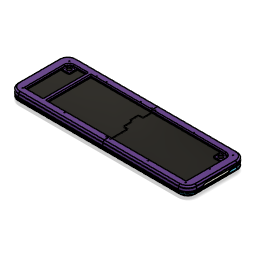
Future Keyboard 2 (Autodesk Fusion 360 design; units mm, degrees)
Autodesk Fusion 360 part; units mm, degrees
note: some values were not read from the file. Chosen so that the rebuilt part matches the saved one: which bodies a step acts on; which face or edge a step refers to; where a step ends. Set by a fixed rule: which sketch regions a step uses.
(part 1 of 2)
sketch "Sketch1" plane through (0, 0, 0) normal (0, 1, 0) x (1, 0, 0)
  arc A0 (365.425, 0) -> (368.425, 3) centre (365.425, 3) ccw
  arc A1 (179.45, 67.614) -> (181.45, 65.614) centre (181.45, 67.614) ccw
  arc A2 (184.212, 48.554) -> (186.212, 46.554) centre (186.212, 48.554) ccw
  circle A3 centre (160.955, 107.775) radius 1.1
  circle A4 centre (363.725, 3.65) radius 1.1
  line L0 (365.425, 111.675) -> (3, 111.675)
  arc A5 (3, 111.675) -> (0, 108.675) centre (3, 108.675) ccw
  circle A6 centre (97.24, 4) radius 1.1
  circle A7 centre (364.375, 55.975) radius 1.1
  line L1 (3, 0) -> (365.425, 0)
  line L2 (368.425, 3) -> (368.425, 108.675)
  circle A8 centre (197.837, 4) radius 1.1
  line L3 (184.212, 63.614) -> (184.212, 48.554)
  line L4 (186.212, 46.554) -> (191.737, 46.554)
  circle A9 centre (184.98, 107.775) radius 1.1
  line L5 (181.45, 65.614) -> (182.212, 65.614)
  circle A10 centre (63.622, 107.775) radius 1.1
  arc A11 (0, 3) -> (3, 0) centre (3, 3) ccw
  arc A12 (181.45, 84.67) -> (179.45, 82.67) centre (181.45, 82.67) ccw
  line L6 (0, 108.675) -> (0, 3)
  circle A13 centre (85.74, 107.775) radius 1.1
  line L7 (186.975, 84.67) -> (181.45, 84.67)
  circle A14 centre (280.925, 4.15) radius 1.1
  arc A15 (184.212, 63.614) -> (182.212, 65.614) centre (182.212, 63.614) ccw
  line L8 (179.45, 82.67) -> (179.45, 67.614)
  arc A16 (193.737, 44.554) -> (191.737, 46.554) centre (191.737, 44.554) ccw
  circle A17 centre (193.075, 107.675) radius 1.1
  circle A18 centre (278.425, 107.625) radius 1.1
  circle A19 centre (4.7, 4.7) radius 1.1
  circle A20 centre (363.825, 107.715) radius 1.1
  arc A21 (368.425, 108.675) -> (365.425, 111.675) centre (365.425, 108.675) ccw
  arc A22 (186.975, 84.67) -> (188.975, 86.67) centre (186.975, 86.67) ccw
  circle A23 centre (4.7, 106.975) radius 1.1
  line L9 (188.975, 111.675) -> (188.975, 86.67)
  line L10 (193.737, 44.554) -> (193.737, 0)
  circle A24 centre (189.74, 4) radius 1.1
  point P0 (368.425, 111.675)
  point P1 (0, 111.675)
  point P2 (184.212, 46.554)
  point P3 (188.975, 84.67)
  point P4 (179.45, 83.9809)
  point P5 (179.45, 65.614)
  point P6 (184.212, 58.87)
  dimension "d1" = 368.425
  dimension "d2" = 111.675
  dimension "d3" = 3
  dimension "d43" = 188.975
  dimension "d45" = 179.45
  dimension "d46" = 184.212
  dimension "d47" = 193.737
  dimension "d48" = 27.005
  dimension "d51" = 2
  dimension "d52" = 19.06
  dimension "d53" = 19.056
  dimension "d227" = 4.7
  dimension "d228" = 4.7
  dimension "d229" = 2.2
  dimension "d230" = 4.7
  dimension "d231" = 3.9
  dimension "d232" = 4
  dimension "d233" = 58.922
  dimension "d234" = 22.118
  dimension "d235" = 75.215
  dimension "d236" = 24.025
  dimension "d237" = 92.54
  dimension "d238" = 92.5
  dimension "d239" = 4
  dimension "d240" = 4.1
  dimension "d242" = 89.45
  dimension "d243" = 3.96
  dimension "d244" = 4.6
  dimension "d245" = 4.05
  dimension "d246" = 55.7
  dimension "d247" = 4.7
  dimension "d248" = 3.65
  dimension "d249" = 87.5
  dimension "d250" = 4.15
  dimension "d251" = 4
  dimension "d252" = 4.1
  dimension "d253" = 4.05
  constraint horizontal L1
  constraint vertical L2
  constraint horizontal L0
  constraint vertical L6
  constraint coincident P1 L0
  constraint coincident P1 L6
  constraint tangent L0 A5
  constraint tangent A5 L6
  constraint coincident origin L1
  constraint coincident origin L6
  constraint tangent L1 A11
  constraint tangent A11 L6
  constraint equal A5 A11
  constraint tangent A0 L1
  constraint tangent A0 L2
  constraint equal A0 A5
  constraint coincident P0 L2
  constraint coincident P0 L0
  constraint tangent L2 A21
  constraint tangent L0 A21
  constraint equal A5 A21
  constraint vertical L9
  constraint coincident L9.start L0
  constraint vertical L8
  constraint vertical L3
  constraint coincident L10.end L1
  constraint perpendicular L1 L10
  constraint perpendicular L7 L9
  constraint perpendicular L5 L8
  constraint perpendicular L4 L10
  constraint coincident P4 L8
  constraint tangent A12 L8
  constraint tangent A12 L7
  constraint coincident P3 L9
  constraint coincident P3 L7
  constraint tangent A22 L9
  constraint tangent L7 A22
  constraint equal A12 A22
  constraint coincident P5 L8
  constraint coincident P5 L5
  constraint tangent A1 L8
  constraint tangent A1 L5
  constraint equal A1 A12
  constraint coincident P6 L3
  constraint tangent L3 A15
  constraint tangent L5 A15
  constraint equal A12 A15
  constraint tangent L4 A16
  constraint tangent A16 L10
  constraint equal A12 A16
  constraint coincident P2 L4
  constraint coincident P2 L3
  constraint tangent A2 L4
  constraint tangent A2 L3
  constraint equal A2 A12
  constraint horizontal A13.centre A3.centre
  constraint horizontal A3.centre A9.centre
  constraint horizontal A6.centre A24.centre
  constraint horizontal A13.centre A10.centre
  constraint equal A10 A23
  constraint equal A10 A13
  constraint equal A3 A13
  constraint equal A3 A9
  constraint equal A9 A24
  constraint equal A6 A24
  constraint equal A6 A19
  constraint vertical A23.centre A19.centre
  constraint equal A17 A18
  constraint equal A18 A20
  constraint equal A7 A20
  constraint equal A4 A7
  constraint equal A4 A14
  constraint equal A8 A14
  constraint equal A3 A17
  constraint coincident L1.start L6
  measures "d1" distance of P0 P1
  measures "d2" distance of origin P1
  measures "d3" radius of A5
  measures "d43" distance of L6 L9
  measures "d45" distance of L6 L8
  measures "d46" distance of L3 L6
  measures "d47" distance of L6 L10
  measures "d48" distance of L9.start P3
  measures "d51" radius of A12
  measures "d52" distance of L4 L5
  measures "d53" distance of L5 L7
  measures "d227" distance of A23.centre L6
  measures "d228" distance of A23.centre L0
  measures "d229" diameter of A23
  measures "d230" distance of A19.centre L1
  measures "d231" distance of A10.centre L0
  measures "d232" distance of A6.centre L1
  measures "d233" horizontal distance of A23.centre A10.centre
  measures "d234" distance of A13.centre A10.centre
  measures "d235" distance of A13.centre A3.centre
  measures "d236" distance of A3.centre A9.centre
  measures "d237" horizontal distance of A19.centre A6.centre
  measures "d238" distance of A6.centre A24.centre
  measures "d239" distance of A17.centre L0
  measures "d240" distance of A17.centre L9
  measures "d242" distance of A18.centre L9
  measures "d243" distance of A20.centre L0
  measures "d244" distance of A20.centre L2
  measures "d245" distance of A7.centre L2
  measures "d246" distance of A7.centre L0
  measures "d247" distance of A4.centre L2
  measures "d248" distance of A4.centre L1
  measures "d249" distance of A14.centre L2
  measures "d250" distance of A14.centre L1
  measures "d251" distance of A8.centre L1
  measures "d252" distance of A8.centre L10
  measures "d253" distance of A18.centre L0
sketch "Sketch2" plane through (0, 0, 0) normal (0, 1, 0) x (1, 0, 0)
  line L0 (360, -8.3249) -> (8.425, -8.3249)
  line L1 (-11.575, 11.6751) -> (-11.575, 99.9999)
  line L2 (8.425, 119.9999) -> (360, 119.9999)
  line L3 (380, 99.9999) -> (380, 11.6751)
  arc A0 (8.425, 119.9999) -> (-11.575, 99.9999) centre (8.425, 99.9999) ccw
  arc A1 (-11.575, 11.6751) -> (8.425, -8.3249) centre (8.425, 11.6751) ccw
  arc A2 (360, -8.3249) -> (380, 11.6751) centre (360, 11.6751) ccw
  arc A3 (380, 99.9999) -> (360, 119.9999) centre (360, 99.9999) ccw
  line L4 (365.425, 111.675) -> (3, 111.675) construction
  line L5 (0, 108.675) -> (0, 3) construction
  line L6 (3, 0) -> (365.425, 0) construction
  line L7 (368.425, 3) -> (368.425, 108.675) construction
  line L8 (0, 55.8375) -> (368.425, 55.8375) construction
  line L9 (184.2125, 0) -> (184.2125, 111.675) construction
  line L10 (8.425, 11.6751) -> (360, 99.9999) construction
  line L11 (8.425, 99.9999) -> (360, 11.6751) construction
  point P0 (3, 3)
  point P1 (3, 108.675)
  point P2 (365.425, 108.675)
  point P3 (365.425, 3)
  point P4 (184.2125, 55.8375)
  dimension "d42" = 20
  constraint horizontal L0
  constraint perpendicular L0 L1
  constraint parallel L0 L2
  constraint parallel L1 L3
  constraint tangent L1 A0
  constraint tangent L2 A0
  constraint tangent L0 A1
  constraint tangent L1 A1
  constraint equal A0 A1
  constraint tangent L0 A2
  constraint tangent L3 A2
  constraint equal A0 A2
  constraint tangent L3 A3
  constraint tangent L2 A3
  constraint equal A0 A3
  constraint midpoint L5 L8.start
  constraint midpoint L7 L8.end
  constraint midpoint L6 L9.start
  constraint midpoint L4 L9.end
  constraint coincident A1.centre L10.start
  constraint coincident A3.centre L10.end
  constraint coincident A0.centre L11.start
  constraint coincident A2.centre L11.end
  constraint midpoint L11 P4
  constraint coincident L9 P4
  constraint coincident L8 P4
  measures "d42" radius of A0
extrude "Extrude3" add sketch "Sketch2" along normal blind 6.6 and the other way blind 20 makes body 1
ref_plane "WorkPlane7" through (184.2125, -20, -55.8375) normal (0, -1, 0) x (-1, 0, 0)
sketch "Sketch3" plane through (-11.575, 0, 0) normal (-1, 0, 0) x (0, 0, 1)
  line L0 (-11.6751, -20) -> (-11.6751, 6.6) construction
  line L1 (-11.6751, 6.6) -> (-99.9999, 6.6) construction
  line L2 (-99.9999, 6.6) -> (-99.9999, -20) construction
  line L3 (-99.9999, -20) -> (-11.6751, -20) construction
  line L4 (-99.9999, -20) -> (-99.9999, 6.6) construction
  line L5 (-99.9999, 6.6) -> (-119.9999, 6.6) construction
  line L6 (-119.9999, 6.6) -> (-119.9999, -20) construction
  line L7 (-119.9999, -20) -> (-99.9999, -20) construction
  line L8 (8.3249, -20) -> (8.3249, 6.6) construction
  line L9 (8.3249, 6.6) -> (-11.6751, 6.6) construction
  line L10 (-11.6751, 6.6) -> (-11.6751, -20) construction
  line L11 (-11.6751, -20) -> (8.3249, -20) construction
  line L12 (8.3249, -20) -> (-119.9999, -20)
  line L13 (-119.9999, -20) -> (8.3249, -13.2748)
  line L14 (8.3249, -13.2748) -> (8.3249, -20)
  dimension "d55" = 3
  constraint coincident L8.start L11.end
  constraint coincident L6.end L7.start
  constraint coincident L8 L13.end
  measures "d55" angle of L12 L13
extrude "Extrude4" cut sketch "Sketch3" against normal through all bodies 1
ref_plane "WorkPlane3" through (184.2125, -13.2748, 8.3249) normal (0, -1, 0) x (1, 0, 0)
ref_plane "WorkPlane4" through (184.2125, -10.2748, 8.3249) normal (0, -1, 0) x (1, 0, 0)
sketch "Sketch4" plane through (184.2125, -10.2748, -55.8375) normal (0, -1, 0) x (1, 0, 0)
  arc A0 (-195.7875, -44.1624) -> (-175.7875, -64.1624) centre (-175.7875, -44.1624) ccw
  line L0 (-175.7875, -64.1624) -> (175.7875, -64.1624)
  arc A1 (175.7875, -64.1624) -> (195.7875, -44.1624) centre (175.7875, -44.1624) ccw
  line L1 (195.7875, -44.1624) -> (195.7875, 44.1624)
  arc A2 (195.7875, 44.1624) -> (175.7875, 64.1624) centre (175.7875, 44.1624) ccw
  line L2 (175.7875, 64.1624) -> (-175.7875, 64.1624)
  arc A3 (-175.7875, 64.1624) -> (-195.7875, 44.1624) centre (-175.7875, 44.1624) ccw
  line L3 (-195.7875, 44.1624) -> (-195.7875, -44.1624)
ref_plane "WorkPlane2" through (184.2125, -6.7, -55.8375) normal (1, 0, 0) x (0, 0, -1)
sketch "Sketch5" plane through (184.2125, -13.9511, -55.8375) normal (1, 0, 0) x (0, 0, -1)
  line L0 (-64.1624, 0.6763) -> (64.1624, -6.0489) construction
  line L1 (64.1624, -6.0489) -> (64.1624, 20.5511) construction
  line L2 (64.1624, 20.5511) -> (-64.1624, 20.5511) construction
  line L3 (-64.1624, 20.5511) -> (-64.1624, 0.6763) construction
  line L4 (64.1624, 3.6763) -> (54.9215, -5.5646)
  line L5 (54.9215, -5.5646) -> (54.1703, -19.8984)
  line L6 (54.1703, -19.8984) -> (81.2796, -21.3191)
  line L7 (81.2796, -21.3191) -> (82.539, 2.7132)
  line L8 (82.539, 2.7132) -> (64.1624, 3.6763)
  point P0 (64.1624, 3.6763)
  dimension "d72" = 45
  constraint coincident P0 L4.start
  constraint coincident L0 L4.end
  constraint perpendicular L0 L5
  constraint perpendicular L5 L6
  constraint perpendicular L6 L7
  constraint perpendicular L5 L8
  measures "d72" angle of L1 L4
sweep "Sweep1" cut profiles "Sketch5" path "Sketch4" along L0 A1 L1 A2 L2 A3 L3 A0 section 1 bodies 1
chamfer "Chamfer1" distance 3 angle 45 8 edges at (-5.7171, 6.6, 2.4671) (184.2125, 6.6, 8.3249) (374.1421, 6.6, 2.4671) (380, 6.6, -55.8375) (374.1421, 6.6, -114.1421) (184.2125, 6.6, -119.9999) (-5.7171, 6.6, -114.1421) (-11.575, 6.6, -55.8375) on bodies 1
ref_plane "WorkPlane5" through (184.2125, 3.6, -55.8375) normal (0, 1, 0) x (1, 0, 0)
ref_plane "WorkPlane6" through (184.2125, -3.3374, -55.8375) normal (0, 1, 0) x (1, 0, 0)
sketch "Sketch6" plane through (0, 0, 0) normal (0, 1, 0) x (1, 0, 0)
  line L0 (8, 85.1196) -> (26.3429, 85.1196)
  line L1 (17.525, 103.4625) -> (46.1, 103.4625)
  line L2 (8, 93.9375) -> (8, 103.4625) construction
  circle A0 centre (17.525, 93.9375) radius 4.5
  line L3 (27.05, 84.4125) -> (27.05, 103.4625) construction
  line L4 (46.1, 8.2125) -> (8, 8.2125)
  line L5 (27.05, 84.4125) -> (8, 103.4625) construction
  arc A1 (17.525, 103.4625) -> (8, 93.9375) centre (17.525, 93.9375) ccw
  line L6 (8, 103.4625) -> (17.525, 103.4625) construction
  line L7 (8, 84.4125) -> (27.05, 103.4625) construction
  line L8 (360.425, 8.2125) -> (55.625, 8.2125)
  line L9 (55.625, 103.4625) -> (350.9, 103.4625)
  arc A2 (360.425, 93.9375) -> (350.9, 103.4625) centre (350.9, 93.9375) ccw
  circle A3 centre (350.9, 93.9375) radius 4.5
  line L10 (341.375, 103.4625) -> (341.375, 84.4125) construction
  line L11 (350.9, 103.4625) -> (360.425, 103.4625) construction
  line L12 (360.425, 103.4625) -> (360.425, 93.9375) construction
  line L13 (342.0821, 103.4625) -> (342.0821, 85.1196)
  circle A4 centre (350.9, 93.9375) radius 7.5 construction
  line L14 (341.375, 103.4625) -> (360.425, 84.4125) construction
  line L15 (342.0821, 85.1196) -> (360.425, 85.1196)
  line L16 (341.375, 84.4125) -> (360.425, 103.4625) construction
  line L17 (360.425, 93.9375) -> (360.425, 8.2125)
  line L18 (341.375, 84.4125) -> (360.425, 84.4125) construction
  line L19 (55.625, 8.2125) -> (55.625, 103.4625)
  line L20 (8, 84.4125) -> (27.05, 84.4125) construction
  line L21 (46.1, 103.4625) -> (46.1, 8.2125)
  line L22 (8, 8.2125) -> (8, 93.9375)
  line L23 (26.3429, 85.1196) -> (26.3429, 103.4625)
  line L24 (365.425, 111.675) -> (3, 111.675)
  line L25 (0, 108.675) -> (0, 3)
  line L26 (3, 0) -> (365.425, 0)
  line L27 (368.425, 3) -> (368.425, 108.675)
  line L28 (360.425, 51.075) -> (368.425, 51.075) construction
  line L29 (0, 55.8375) -> (8, 55.8375) construction
  line L30 (184.2125, 0) -> (184.2125, 8.2125) construction
  line L31 (184.2125, 111.675) -> (184.2125, 103.4625) construction
  line L32 (24.525, 100.9375) -> (10.525, 100.9375)
  line L33 (10.525, 100.9375) -> (10.525, 86.9375)
  line L34 (10.525, 86.9375) -> (24.525, 86.9375)
  line L35 (24.525, 86.9375) -> (24.525, 100.9375)
  line L36 (24.525, 100.9375) -> (10.525, 86.9375) construction
  line L37 (10.525, 100.9375) -> (24.525, 86.9375) construction
  line L38 (357.9, 100.9375) -> (343.9, 100.9375)
  line L39 (343.9, 100.9375) -> (343.9, 86.9375)
  line L40 (343.9, 86.9375) -> (357.9, 86.9375)
  line L41 (357.9, 86.9375) -> (357.9, 100.9375)
  line L42 (357.9, 100.9375) -> (343.9, 86.9375) construction
  line L43 (343.9, 100.9375) -> (357.9, 86.9375) construction
  point P0 (191.1727, 8.2125)
  point P1 (8, 59.175)
  point P2 (360.425, 54.8137)
  point P3 (17.525, 93.9375)
  point P4 (350.9, 93.9375)
  dimension "d185" = -1
  dimension "d186" = -1
  dimension "d7" = 304.8
  dimension "d8" = 95.25
  dimension "d9" = 38.1
  dimension "d10" = 9.525
  dimension "d176" = 19.05
  dimension "d177" = 15
  dimension "d180" = 19.05
  dimension "d181" = 9
  dimension "d182" = 9
  dimension "d87" = 1
  dimension "d198" = 14
  dimension "d199" = 14
  constraint coincident P0 L8
  constraint equal L19 L21
  constraint collinear L1 L9
  constraint coincident P1 L22
  constraint coincident L10.start L9
  constraint perpendicular L9 L10
  constraint coincident L14.end L17
  constraint perpendicular L17 L18
  constraint equal L10 L18
  constraint midpoint P4 L16
  constraint concentric A2 A4
  constraint tangent L9 A2
  constraint coincident P2 L17
  constraint tangent L1 A1
  constraint tangent A1 L22
  constraint equal A1 A2
  constraint coincident L7.start L22
  constraint perpendicular L20 L22
  constraint coincident L3.end L1
  constraint perpendicular L1 L3
  constraint equal L3 L20
  constraint concentric A3 A4
  constraint concentric A0 A1
  constraint parallel L0 L20
  constraint parallel L3 L23
  constraint parallel L10 L13
  constraint parallel L15 L18
  constraint midpoint L17 L28.start
  constraint coincident L27 L28.end
  constraint perpendicular L27 L28
  constraint midpoint L25 L29.start
  constraint coincident L22 L29.end
  constraint perpendicular L22 L29
  constraint perpendicular L8 L17
  constraint perpendicular L8 L19
  constraint perpendicular L9 L19
  constraint perpendicular L4 L21
  constraint perpendicular L4 L22
  constraint coincident L23.end L1
  constraint coincident L0.start L22
  constraint coincident L0.end L5
  constraint perpendicular L2 L6
  constraint perpendicular L3 L6
  constraint midpoint L26 L30.start
  constraint coincident L8 L30.end
  constraint perpendicular L8 L30
  constraint midpoint L24 L31.start
  constraint coincident L9 L31.end
  constraint perpendicular L9 L31
  constraint equal L30 L31
  constraint parallel L9 L24
  constraint coincident L13.end L16
  constraint coincident L13.start L9
  constraint coincident L15.end L17
  constraint tangent A2 L17
  constraint equal L28 L29
  constraint perpendicular L11 L12
  constraint equal L0 L15
  constraint horizontal L32
  constraint perpendicular L32 L33
  constraint parallel L32 L34
  constraint parallel L33 L35
  constraint coincident L7 L32.start
  constraint coincident L36 P3
  constraint coincident L37 P3
  constraint coincident P3 A0.centre
  constraint horizontal L38
  constraint perpendicular L38 L39
  constraint parallel L38 L40
  constraint parallel L39 L41
  constraint coincident L16 L38.start
  constraint coincident L42 P4
  constraint coincident L43 P4
  constraint coincident P4 A2.centre
  measures "d7" distance of L9.start L11.end
  measures "d8" distance of L9.start L8.end
  measures "d9" distance of L2.end L1.end
  measures "d10" distance of L19 L21
  measures "d176" distance of L10.start L10.end
  measures "d177" diameter of A4
  measures "d180" distance of L3.start L3.end
  measures "d181" diameter of A3
  measures "d182" diameter of A0
  measures "d87" distance of L0.end L3.start
  measures "d198" distance of L32.start L32.end
  measures "d199" distance of L38.start L38.end
extrude "Extrude5" cut sketch "Sketch6" along normal through all contours L0 L1 L4 L21 L22 L23 | L8 L9 L13 L15 L17 L19 bodies 1
extrude "Extrude6" cut sketch "Sketch1" along normal blind 1.6 contours A0 A1 A2 L0 L1 L2 L3 L4 L5 A12 L7 A15 L8 A16 A21 A22 L9 L10 | A1 A2 L0 A5 L1 L3 L4 L5 A11 A12 L6 L7 A15 L8 A16 A22 L9 L10 | A3 | A4 | A6 | A7 | A8 | A9 | A10 | A13 | A14 | A17 | A18 | A19 | A20 | A23 | A24 bodies 1
extrude "Extrude10" add sketch "Sketch1" along normal blind 1.6 separate body makes body 2
extrude "Extrude8" cut sketch "Sketch6" along normal through all contours A0 | A3 bodies 1
extrude "Extrude9" cut sketch "Sketch6" against normal blind 3 from surface at 6.6 contours L0 L1 A1 L22 L23 L32 L33 L34 L35 | A1 L32 L33 L34 L35 | L9 A2 L13 L15 L17 L38 L39 L40 L41 | A2 L38 L39 L40 L41 bodies 1
extrude "Extrude23" cut sketch "Sketch6" along normal blind 1 from surface at 1.6 contours A1 L32 L33 | A1 L32 L33 L34 L35 | A2 L38 L39 L40 L41 | A2 L38 L41 bodies 1
chamfer "Chamfer2" distance 2 angle 45 2 edges at (342.0821, 2.6, -85.1196) (26.3429, 2.6, -85.1196) on bodies 1
chamfer "Chamfer3" distance 2 angle 45 10 edges at (31.8125, 6.6, -103.4625) (8, 6.6, -51.075) (10.7898, 6.6, -100.6727) (46.1, 6.6, -55.8375) (27.05, 6.6, -8.2125) (55.625, 6.6, -55.8375) (203.2625, 6.6, -103.4625) (357.6352, 6.6, -100.6727) (360.425, 6.6, -51.075) (208.025, 6.6, -8.2125) on bodies 1
split "Split1" by plane through (0, 0, 0) normal (0, 1, 0) bodies 1 makes body 3 at (372.1417, 6.6, -68.5375)
shell "Shell1" thickness 5 removed faces 2 at (244.6167, 0, -37.225) at (372.2833, 0, -70.5583) on bodies 1
sketch "Sketch7" plane through (184.2125, -9.2, -55.8375) normal (1, 0, 0) x (0, 0, -1)
  line L0 (159.4764, 5.8626) -> (-230.5357, 5.8626) construction
  line L1 (-60.9965, -4.2407) -> (54.9215, -10.3157) construction
  line L2 (54.9215, -10.3157) -> (64.1624, -1.0748) construction
  line L3 (64.1624, -1.0748) -> (64.1624, 9.2) construction
  line L4 (64.1624, 9.2) -> (59.1624, 9.2) construction
  line L5 (59.1624, 9.2) -> (59.1624, 0.9963) construction
  line L6 (59.1624, 0.9963) -> (52.9601, -5.206) construction
  line L7 (52.9601, -5.206) -> (-58.8181, 0.652) construction
  line L8 (-58.8181, 0.652) -> (-59.1624, 0.9963) construction
  line L9 (-59.1624, 0.9963) -> (-59.1624, 9.2) construction
  line L10 (-59.1624, 9.2) -> (-64.1624, 9.2) construction
  line L11 (-64.1624, 9.2) -> (-64.1624, -1.0748) construction
  line L12 (-64.1624, -1.0748) -> (-60.9965, -4.2407) construction
  line L13 (-64.1624, 5.8626) -> (-64.1624, 8.8626) construction
  line L14 (-64.1624, 8.8626) -> (-59.1624, 8.8626) construction
  line L15 (-59.1624, 8.8626) -> (-59.1624, 2.8626) construction
  line L16 (-64.1624, 2.8626) -> (-59.1624, 2.8626) construction
  line L17 (-64.1624, 2.8626) -> (-64.1624, 5.8626) construction
  line L18 (-64.1624, 5.8626) -> (-64.1624, 8.8626)
  line L19 (-64.1624, 8.8626) -> (-63.0134, 8.8626)
  line L20 (-63.0134, 8.8626) -> (-63.0134, 10.8626)
  line L21 (-63.0134, 10.8626) -> (-61.4134, 10.8626)
  line L22 (-61.4134, 10.8626) -> (-61.4134, 8.8626)
  line L23 (-64.1624, 2.8626) -> (-63.0134, 2.8626)
  line L24 (-63.0134, 0.8626) -> (-61.4134, 0.8626)
  line L25 (-61.4134, 0.8626) -> (-61.4134, 2.8626)
  line L26 (-63.0134, 2.8626) -> (-63.0134, 0.8626)
  line L27 (-61.4134, 2.8626) -> (-59.1624, 2.8626)
  line L28 (-59.1624, 2.8626) -> (-59.1624, 8.8626)
  line L29 (-59.1624, 8.8626) -> (-61.4134, 8.8626)
  line L30 (-64.1624, 5.8626) -> (-64.1624, 2.8626)
  line L31 (-63.0134, 8.8626) -> (-63.0134, 2.8626)
  line L32 (-61.4134, 2.8626) -> (-61.4134, 8.8626)
  line L33 (-61.2134, 11.0626) -> (-61.2134, 8.8626)
  line L34 (-61.2134, 2.8626) -> (-61.2134, 8.8626)
  line L35 (-61.2134, 0.6626) -> (-61.2134, 2.8626)
  line L36 (-63.2134, 0.6626) -> (-61.2134, 0.6626)
  line L37 (-63.2134, 2.8626) -> (-63.2134, 0.6626)
  line L38 (-63.2134, 8.8626) -> (-63.2134, 2.8626)
  line L39 (-63.2134, 8.8626) -> (-63.2134, 11.0626)
  line L40 (-63.2134, 11.0626) -> (-61.2134, 11.0626)
  dimension "d92" = 3
  dimension "d93" = 1.6
  dimension "d134" = 2
  constraint coincident L11 L13.start
  constraint coincident L0 L13.start
  constraint perpendicular L0 L13
  constraint coincident L9 L14.end
  constraint perpendicular L9 L14
  constraint coincident L9 L15.end
  constraint perpendicular L0 L15
  constraint coincident L11 L16.start
  constraint perpendicular L15 L16
  constraint perpendicular L0 L17
  constraint equal L13 L17
  constraint coincident L14 L19.end
  constraint perpendicular L19 L20
  constraint perpendicular L20 L21
  constraint coincident L14 L22.end
  constraint perpendicular L14 L22
  constraint coincident L16 L23.end
  constraint perpendicular L11 L23
  constraint perpendicular L11 L24
  constraint coincident L16 L25.end
  constraint perpendicular L16 L25
  constraint perpendicular L24 L26
  constraint equal L21 L24
  constraint equal L20 L26
  constraint equal L19 L23
  measures "d92" distance of L13.start L13.end
  measures "d93" distance of L20.end L21.end
  measures "d134" distance of L19.end L20.end
sweep "Sweep2" cut profiles "Sketch7" path "Sketch4" along A1 L1 A2 L2 A3 L3 A0 L0 section 1 contours L19 L20 L21 L22 L29 L33 L39 L40 | L19 L23 L31 L38 | L23 L24 L25 L26 L27 L35 L36 L37 | L20 L21 L22 L24 L25 L26 L31 L32 | L27 L29 L32 L34 bodies 3 1
sweep "Sweep3" add profiles "Sketch7" path "Sketch4" along L3 A0 L0 A1 L1 A2 L2 A3 section 1 contours L20 L21 L22 L24 L25 L26 L31 L32 separate body makes body 4
combine "Combine1" operation add target body 3 tool bodies 1
sketch "Sketch8" plane through (-11.575, 0, 0) normal (-1, 0, 0) x (0, 0, 1)
  line L0 (-11.6751, -10.2748) -> (-11.6751, 3.6)
  line L1 (-11.6751, 3.6) -> (-99.9999, 3.6)
  line L2 (-99.9999, 3.6) -> (-99.9999, -10.2748)
  line L3 (-99.9999, -10.2748) -> (-11.6751, -10.2748)
  line L4 (-110.759, -19.5157) -> (-99.9999, -18.9518)
  line L5 (-99.9999, -18.9518) -> (-11.6751, -14.3229)
  line L6 (-11.6751, -14.3229) -> (5.159, -13.4407)
  line L7 (-119.9999, -10.2748) -> (-110.759, -19.5157)
  line L8 (8.3249, -10.2748) -> (5.159, -13.4407)
  line L9 (8.3249, 3.6) -> (8.3249, -10.2748)
  line L10 (8.3249, 3.6) -> (5.3249, 6.6)
  line L11 (-11.6751, 6.6) -> (5.3249, 6.6)
  line L12 (-99.9999, 6.6) -> (-11.6751, 6.6)
  line L13 (-119.9999, 3.6) -> (-116.9999, 6.6)
  line L14 (-116.9999, 6.6) -> (-99.9999, 6.6)
  line L15 (-119.9999, -10.2748) -> (-119.9999, 3.6)
  line L16 (-119.9999, 3.6) -> (8.3249, 3.6)
  line L17 (8.3249, -10.2748) -> (-119.9999, -10.2748)
  line L18 (8.3249, -6.3374) -> (-80.4619, -6.3374)
  line L19 (-119.9999, -0.3374) -> (-31.2131, -0.3374)
  line L20 (-82.9619, -5.6675) -> (-85.8375, -4.0073)
  line L21 (-119.9999, -3.3374) -> (-88.3375, -3.3374)
  line L22 (-28.7131, -1.0073) -> (-25.8375, -2.6675)
  line L23 (-23.3375, -3.3374) -> (8.3249, -3.3374)
  arc A0 (-85.8375, -4.0073) -> (-88.3375, -3.3374) centre (-88.3375, -8.3374) ccw
  arc A1 (-82.9619, -5.6675) -> (-80.4619, -6.3374) centre (-80.4619, -1.3374) ccw
  arc A2 (-28.7131, -1.0073) -> (-31.2131, -0.3374) centre (-31.2131, -5.3374) ccw
  arc A3 (-25.8375, -2.6675) -> (-23.3375, -3.3374) centre (-23.3375, 1.6626) ccw
  dimension "d110" = 5
  dimension "d129" = 65
  dimension "d130" = 3
  dimension "d131" = 3
  dimension "d132" = 30
  constraint coincident L13.start L15.end
  constraint coincident L9.start L10.start
  constraint coincident L8.start L9.end
  constraint coincident L7.start L15.start
  constraint coincident L9 L18.start
  constraint perpendicular L9 L18
  constraint coincident L15 L19.start
  constraint perpendicular L15 L19
  constraint midpoint L9 L23.end
  constraint coincident L15 L21.start
  constraint midpoint L15 L21.start
  constraint tangent L20 A0
  constraint tangent L21 A0
  constraint tangent L18 A1
  constraint tangent L20 A1
  constraint equal A0 A1
  constraint tangent L19 A2
  constraint tangent L22 A2
  constraint equal A0 A2
  constraint tangent L22 A3
  constraint tangent L23 A3
  constraint equal A0 A3
  constraint perpendicular L15 L21
  constraint parallel L16 L23
  constraint equal L20 L22
  constraint equal L21 L23
  constraint parallel L20 L22
  measures "d110" radius of A0
  measures "d129" distance of L21.end L23.start
  measures "d130" distance of L19.start L21.start
  measures "d131" distance of L18.start L23.end
  measures "d132" angle of L20 L21
extrude "Extrude7" cut sketch "Sketch8" against normal through all contours L0 L2 L18 L19 L20 L21 L22 L23 A0 A1 A2 A3 | L0 L9 L18 L23 | L2 L15 L19 L21 bodies 3 makes body 5 at (372.1417, 6.6, -68.5375)
sketch "Sketch9" plane through (0, 0, 0) normal (0, 1, 0) x (1, 0, 0)
  arc A0 (186.975, 84.67) -> (188.975, 86.67) centre (186.975, 86.67) ccw
  line L0 (186.975, 84.67) -> (181.45, 84.67)
  arc A1 (181.45, 84.67) -> (179.45, 82.67) centre (181.45, 82.67) ccw
  line L1 (179.45, 82.67) -> (179.45, 67.614)
  arc A2 (179.45, 67.614) -> (181.45, 65.614) centre (181.45, 67.614) ccw
  line L2 (181.45, 65.614) -> (182.212, 65.614)
  arc A3 (184.212, 63.614) -> (182.212, 65.614) centre (182.212, 63.614) ccw
  line L3 (184.212, 63.614) -> (184.212, 48.554)
  arc A4 (184.212, 48.554) -> (186.212, 46.554) centre (186.212, 48.554) ccw
  line L4 (186.212, 46.554) -> (191.737, 46.554)
  arc A5 (193.737, 44.554) -> (191.737, 46.554) centre (191.737, 44.554) ccw
  line L5 (193.737, 44.554) -> (193.737, 0)
  line L6 (188.975, 111.675) -> (188.975, 86.67)
  line L7 (365.425, 111.675) -> (3, 111.675) construction
  line L8 (3, 0) -> (365.425, 0) construction
  line L9 (187.175, 111.675) -> (187.175, 86.67)
  arc A6 (186.975, 86.47) -> (187.175, 86.67) centre (186.975, 86.67) ccw
  line L10 (186.975, 86.47) -> (181.45, 86.47)
  arc A7 (181.45, 86.47) -> (177.65, 82.67) centre (181.45, 82.67) ccw
  line L11 (177.65, 82.67) -> (177.65, 67.614)
  arc A8 (177.65, 67.614) -> (181.45, 63.814) centre (181.45, 67.614) ccw
  line L12 (181.45, 63.814) -> (182.212, 63.814)
  arc A9 (182.412, 63.614) -> (182.212, 63.814) centre (182.212, 63.614) ccw
  line L13 (182.412, 63.614) -> (182.412, 48.554)
  arc A10 (182.412, 48.554) -> (186.212, 44.754) centre (186.212, 48.554) ccw
  line L14 (186.212, 44.754) -> (191.737, 44.754)
  arc A11 (191.937, 44.554) -> (191.737, 44.754) centre (191.737, 44.554) ccw
  line L15 (191.937, 44.554) -> (191.937, 0)
  line L16 (190.775, 111.675) -> (190.775, 86.67)
  arc A12 (186.975, 82.87) -> (190.775, 86.67) centre (186.975, 86.67) ccw
  line L17 (186.975, 82.87) -> (181.45, 82.87)
  arc A13 (181.45, 82.87) -> (181.25, 82.67) centre (181.45, 82.67) ccw
  line L18 (181.25, 82.67) -> (181.25, 67.614)
  arc A14 (181.25, 67.614) -> (181.45, 67.414) centre (181.45, 67.614) ccw
  line L19 (181.45, 67.414) -> (182.212, 67.414)
  arc A15 (186.012, 63.614) -> (182.212, 67.414) centre (182.212, 63.614) ccw
  line L20 (186.012, 63.614) -> (186.012, 48.554)
  arc A16 (186.012, 48.554) -> (186.212, 48.354) centre (186.212, 48.554) ccw
  line L21 (186.212, 48.354) -> (191.737, 48.354)
  arc A17 (195.537, 44.554) -> (191.737, 48.354) centre (191.737, 44.554) ccw
  line L22 (195.537, 44.554) -> (195.537, 0)
  line L23 (191.937, 0) -> (191.937, -5.3759)
  line L24 (195.537, 0) -> (195.537, -5.3759)
  line L25 (187.175, 111.675) -> (187.175, 117.0509)
  line L26 (190.775, 111.675) -> (190.775, 117.0509)
  line L27 (8.425, 117.0509) -> (360, 117.0509)
  line L28 (360, -5.3759) -> (8.425, -5.3759)
  dimension "d119" = 1.8
  dimension "d120" = -1.8
  constraint perpendicular L7 L25
  constraint coincident L24.end L28
  constraint coincident L23.end L28
  constraint collinear L15 L23
  constraint collinear L22 L24
  constraint coincident L26.end L27
  constraint coincident L25.end L27
  constraint collinear L16 L26
extrude "Extrude11" add sketch "Sketch9" along normal up to near side of body 3 bodies 3
sketch "Sketch10" plane through (195.537, 0, 0) normal (1, 0, 0) x (0, 0, -1)
  line L0 (-2.9806, -8.548) -> (44.554, -11.0392)
  line L1 (44.554, -11.0392) -> (44.554, 0)
  line L2 (44.554, 0) -> (-5.3759, 0)
  line L3 (-5.3759, -6.3374) -> (-3.3249, -6.3374)
  line L4 (-3.3249, -8.2037) -> (-2.9806, -8.548)
  line L5 (8.2125, 4.6) -> (6.2125, 6.6)
  line L6 (6.2125, 6.6) -> (-5.3249, 6.6)
  line L7 (-5.3249, 6.6) -> (-8.3249, 3.6)
  line L8 (-8.3249, 3.6) -> (-8.3249, -3.3374)
  line L9 (-8.3249, -3.3374) -> (-7.3759, -3.3374)
  line L10 (-5.3759, -3.3374) -> (-3.3249, -3.3374)
  line L11 (-3.3249, -3.3374) -> (-3.3249, 0)
  line L12 (-3.3249, 0) -> (0, 0)
  line L13 (0, 0) -> (0, 1.6)
  line L14 (0, 1.6) -> (8.2125, 1.6)
  line L15 (8.2125, 1.6) -> (8.2125, 4.6)
  line L16 (105.4625, 6.6) -> (103.4625, 4.6)
  line L17 (103.4625, 4.6) -> (103.4625, 1.6)
  line L18 (103.4625, 1.6) -> (111.675, 1.6)
  line L19 (111.675, 1.6) -> (111.675, 0)
  line L20 (111.675, 0) -> (114.9999, 0)
  line L21 (119.9999, -0.3374) -> (119.9999, 3.6)
  line L22 (119.9999, 3.6) -> (116.9999, 6.6)
  line L23 (116.9999, 6.6) -> (105.4625, 6.6)
  line L24 (-5.3759, 0) -> (-3.1249, 0)
  line L25 (-3.1249, 0) -> (-3.1249, -3.1374)
  line L26 (-3.1249, -3.1374) -> (-5.3759, -3.1374)
  line L27 (-5.3759, -3.1374) -> (-5.3759, 0)
  line L28 (86.67, -13.2464) -> (108.7976, -14.406)
  line L29 (108.7976, -14.406) -> (114.9999, -8.2037)
  line L30 (114.9999, -8.2037) -> (114.9999, -3.3374)
  line L31 (114.9999, -3.3374) -> (117.0509, -3.3374)
  line L32 (117.0509, 0) -> (86.67, 0)
  line L33 (86.67, 0) -> (86.67, -13.2464)
  line L34 (117.0509, 0) -> (114.7999, 0)
  line L35 (114.7999, 0) -> (114.7999, -0.5374)
  line L36 (114.7999, -0.5374) -> (117.0509, -0.5374)
  line L37 (117.0509, -0.5374) -> (117.0509, 0)
  line L38 (-3.3249, -6.3374) -> (-3.3249, -8.2037)
  line L39 (-5.3759, 0) -> (-5.3759, -6.3374)
  line L40 (114.9999, 0) -> (114.9999, -0.3374)
  line L41 (114.9999, -0.3374) -> (117.0509, -0.3374)
  line L42 (117.0509, -0.3374) -> (117.0509, 1.8626)
  line L43 (117.0509, 1.8626) -> (119.0509, 1.8626)
  line L44 (119.0509, 1.8626) -> (119.0509, -0.3374)
  line L45 (119.0509, -0.3374) -> (119.9999, -0.3374)
  line L46 (-7.3759, -3.3374) -> (-7.3759, 1.8626)
  line L47 (-7.3759, 1.8626) -> (-5.3759, 1.8626)
  line L48 (-5.3759, 1.8626) -> (-5.3759, -3.3374)
  line L49 (117.0509, -3.3374) -> (117.0509, 0)
  dimension "d124" = 0.2
  dimension "d125" = 0.2
  dimension "d126" = 0.2
  dimension "d203" = 0.2
  constraint horizontal L24
  constraint vertical L25
  constraint horizontal L26
  constraint vertical L27
  constraint coincident L2.end L24.start
  constraint horizontal L34
  constraint vertical L35
  constraint horizontal L36
  constraint vertical L37
  constraint coincident L32.start L34.start
  measures "d124" distance of L11 L25
  measures "d125" distance of L10.start L26.end
  measures "d126" distance of L20.end L34.end
  measures "d203" distance of L36 L41
extrude "Extrude12" cut sketch "Sketch10" against normal through all contours L2 L11 L12 L24 L25 L26 | L2 L11 L24 L26 L27 L39 L48 | L20 L32 L34 L35 L36 L37 L40 L41 L49 | L32 L34 L37 L40 L41 L42 L49 bodies 3
copy_body "CopyPasteBodies1" bodies 3 makes body 6
move_body "Move1" bodies 6 to x (1, 0, 0) y (0, 1, 0) z (0, 0, 1) at (0, 0, 0)
combine "Combine2" operation cut target body 5 tool bodies 6
split "Split2" by curves path "Sketch1" along L9 A22 L7 A12 L8 A1 L5 A15 L3 A2 L4 A16 L10 bodies 2 3 4 5 makes body 10 at (-3.7167, 6.6, -68.5375) makes body 9 at (70.1957, -2.3374, 7.1759) makes body 8 at (65.4333, -16.737, -57.738) makes body 7 at (121.2224, 0, -59.7458)
sketch "Sketch11" plane through (0, 0, 0) normal (0, 1, 0) x (1, 0, 0)
  circle A0 centre (4.7, 106.975) radius 1.1 construction
  circle A1 centre (63.622, 107.775) radius 1.1 construction
  circle A2 centre (85.74, 107.775) radius 1.1 construction
  circle A3 centre (97.24, 4) radius 1.1 construction
  circle A4 centre (189.74, 4) radius 1.1 construction
  circle A5 centre (184.98, 107.775) radius 1.1 construction
  circle A6 centre (160.955, 107.775) radius 1.1 construction
  circle A7 centre (193.075, 107.675) radius 1.1 construction
  circle A8 centre (197.837, 4) radius 1.1 construction
  circle A9 centre (280.925, 4.15) radius 1.1 construction
  circle A10 centre (278.425, 107.625) radius 1.1 construction
  circle A11 centre (363.825, 107.715) radius 1.1 construction
  circle A12 centre (364.375, 55.975) radius 1.1 construction
  circle A13 centre (363.725, 3.65) radius 1.1 construction
  circle A14 centre (4.7, 4.7) radius 1.1 construction
  circle A15 centre (4.7, 106.975) radius 3.5
  circle A16 centre (4.7, 106.975) radius 1.2
  circle A17 centre (63.622, 107.775) radius 1.2
  circle A18 centre (63.622, 107.775) radius 3.5
  circle A19 centre (85.74, 107.775) radius 1.2
  circle A20 centre (85.74, 107.775) radius 3.5
  circle A21 centre (160.955, 107.775) radius 1.2
  circle A22 centre (160.955, 107.775) radius 3.5
  circle A23 centre (184.98, 107.775) radius 1.2
  circle A24 centre (184.98, 107.775) radius 3.5
  circle A25 centre (193.075, 107.675) radius 1.2
  circle A26 centre (193.075, 107.675) radius 3.5
  circle A27 centre (278.425, 107.625) radius 1.2
  circle A28 centre (278.425, 107.625) radius 3.5
  circle A29 centre (363.825, 107.715) radius 1.2
  circle A30 centre (363.825, 107.715) radius 3.5
  circle A31 centre (364.375, 55.975) radius 1.2
  circle A32 centre (364.375, 55.975) radius 3.5
  circle A33 centre (363.725, 3.65) radius 1.2
  circle A34 centre (363.725, 3.65) radius 3.5
  circle A35 centre (280.925, 4.15) radius 1.2
  circle A36 centre (280.925, 4.15) radius 3.5
  circle A37 centre (197.837, 4) radius 1.2
  circle A38 centre (197.837, 4) radius 3.5
  circle A39 centre (189.74, 4) radius 1.2
  circle A40 centre (189.74, 4) radius 3.5
  circle A41 centre (97.24, 4) radius 1.2
  circle A42 centre (97.24, 4) radius 3.5
  circle A43 centre (4.7, 4.7) radius 1.2
  circle A44 centre (4.7, 4.7) radius 3.5
  dimension "d142" = 2.4
  dimension "d143" = 7
  constraint concentric A0 A15
  constraint concentric A15 A16
  constraint concentric A1 A17
  constraint concentric A17 A18
  constraint concentric A2 A19
  constraint concentric A2 A20
  constraint concentric A6 A21
  constraint concentric A21 A22
  constraint concentric A5 A23
  constraint concentric A5 A24
  constraint concentric A7 A25
  constraint concentric A7 A26
  constraint concentric A10 A27
  constraint concentric A10 A28
  constraint concentric A11 A29
  constraint concentric A11 A30
  constraint concentric A12 A31
  constraint concentric A12 A32
  constraint concentric A13 A33
  constraint concentric A33 A34
  constraint concentric A9 A35
  constraint concentric A9 A36
  constraint concentric A8 A37
  constraint concentric A37 A38
  constraint concentric A4 A39
  constraint concentric A4 A40
  constraint concentric A3 A42
  constraint concentric A14 A43
  constraint concentric A43 A44
  constraint equal A16 A17
  constraint equal A17 A19
  constraint equal A19 A21
  constraint equal A21 A23
  constraint equal A23 A25
  constraint equal A25 A27
  constraint equal A27 A29
  constraint equal A29 A31
  constraint equal A31 A33
  constraint equal A33 A35
  constraint equal A35 A37
  constraint equal A37 A39
  constraint equal A39 A41
  constraint equal A41 A43
  constraint equal A15 A18
  constraint equal A15 A20
  constraint equal A20 A22
  constraint equal A22 A26
  constraint equal A24 A26
  constraint equal A24 A28
  constraint equal A28 A30
  constraint equal A30 A32
  constraint equal A32 A34
  constraint equal A34 A36
  constraint equal A36 A40
  constraint equal A38 A40
  constraint equal A38 A42
  constraint equal A42 A44
  constraint coincident A3.centre A41.centre
  measures "d142" diameter of A16
  measures "d143" diameter of A15
extrude "Extrude15" cut sketch "Sketch11" against normal through all contours A16 | A17 | A19 | A21 | A23 | A25 | A27 | A29 | A31 | A33 | A35 | A37 | A39 | A41 | A43 bodies 3 8
extrude "Extrude14" add sketch "Sketch11" along normal up to near side of body 8 contours A15 | A18 | A20 | A22 | A24 | A40 | A42 | A44 bodies 8
extrude "Extrude16" add sketch "Sketch11" along normal up to near side of body 3 contours A26 | A28 | A30 | A32 | A34 | A36 | A38 bodies 3
sketch "Sketch12" plane through (0, 0, 0) normal (0, 1, 0) x (1, 0, 0)
  circle A0 centre (4.7, 106.975) radius 1.375
  circle A1 centre (63.622, 107.775) radius 1.375
  circle A2 centre (85.74, 107.775) radius 1.375
  circle A3 centre (160.955, 107.775) radius 1.375
  circle A4 centre (184.98, 107.775) radius 1.375
  circle A5 centre (193.075, 107.675) radius 1.375
  circle A6 centre (278.425, 107.625) radius 1.375
  circle A7 centre (363.825, 107.715) radius 1.375
  circle A8 centre (364.375, 55.975) radius 1.375
  circle A9 centre (363.725, 3.65) radius 1.375
  circle A10 centre (280.925, 4.15) radius 1.375
  circle A11 centre (197.837, 4) radius 1.375
  circle A12 centre (189.74, 4) radius 1.375
  circle A13 centre (97.24, 4) radius 1.375
  circle A14 centre (4.7, 4.7) radius 1.375
  point P0 (363.725, 3.65)
  point P1 (364.375, 55.975)
  point P2 (363.825, 107.715)
  point P3 (278.425, 107.625)
  point P4 (280.925, 4.15)
  point P5 (197.837, 4)
  point P6 (189.74, 4)
  point P7 (97.24, 4)
  point P8 (4.7, 4.7)
  point P9 (63.622, 107.775)
  point P10 (85.74, 107.775)
  point P11 (160.955, 107.775)
  point P12 (184.98, 107.775)
  point P13 (193.075, 107.675)
  point P14 (4.7, 106.975)
  dimension "d139" = 2.75
  constraint coincident P14 A0.centre
  constraint coincident P9 A1.centre
  constraint coincident P10 A2.centre
  constraint coincident P11 A3.centre
  constraint coincident P12 A4.centre
  constraint coincident P13 A5.centre
  constraint coincident P3 A6.centre
  constraint coincident P2 A7.centre
  constraint coincident P0 A9.centre
  constraint coincident P1 A8.centre
  constraint coincident P4 A10.centre
  constraint coincident P5 A11.centre
  constraint coincident P6 A12.centre
  constraint coincident P7 A13.centre
  constraint coincident P8 A14.centre
  constraint equal A0 A1
  constraint equal A1 A2
  constraint equal A2 A3
  constraint equal A3 A5
  constraint equal A4 A5
  constraint equal A4 A6
  constraint equal A6 A7
  constraint equal A7 A8
  constraint equal A8 A9
  constraint equal A9 A10
  constraint equal A10 A11
  constraint equal A11 A12
  constraint equal A12 A13
  constraint equal A13 A14
  measures "d139" diameter of A0
extrude "Extrude13" cut sketch "Sketch12" along normal blind 5.6 bodies 5 10
sketch "Sketch13" plane through (184.2125, -20, -55.8375) normal (0, -1, 0) x (1, 0, 0)
  circle A0 centre (0.7675, -51.9375) radius 1.2 construction
  line L0 (-175.7875, -54.9215) -> (4.7625, -54.9215) construction
  line L1 (4.7625, -54.9215) -> (4.7625, -30.8325) construction
  arc A1 (4.7625, -30.8325) -> (2.7625, -28.8325) centre (2.7625, -30.8325) ccw construction
  line L2 (2.7625, -28.8325) -> (-2.7625, -28.8325) construction
  arc A2 (-4.7625, -26.8325) -> (-2.7625, -28.8325) centre (-2.7625, -26.8325) ccw construction
  line L3 (-4.7625, -26.8325) -> (-4.7625, -11.7765) construction
  arc A3 (-2.7625, -9.7765) -> (-4.7625, -11.7765) centre (-2.7625, -11.7765) ccw construction
  line L4 (-2.7625, -9.7765) -> (-2.0005, -9.7765) construction
  arc A4 (-2.0005, -9.7765) -> (-0.0005, -7.7765) centre (-2.0005, -7.7765) ccw construction
  line L5 (-0.0005, -7.7765) -> (-0.0005, 7.2835) construction
  arc A5 (1.9995, 9.2835) -> (-0.0005, 7.2835) centre (1.9995, 7.2835) ccw construction
  line L6 (1.9995, 9.2835) -> (7.5245, 9.2835) construction
  arc A6 (7.5245, 9.2835) -> (9.5245, 11.2835) centre (7.5245, 11.2835) ccw construction
  line L7 (9.5245, 11.2835) -> (9.5245, 60.9965) construction
  line L8 (9.5245, 60.9965) -> (-175.7875, 60.9965) construction
  ellipse E0 centre (-175.7875, 45.0007) end of major axis (-175.7875, 60.9965) minor radius 15.9738 (-175.7875, 60.9965) -> (-191.7393, 44.1624) ccw
  line L9 (-191.7393, 44.1624) -> (-187.1104, -44.1624) construction
  ellipse E1 centre (-175.7875, -43.5674) end of major axis (-175.7875, -54.9215) minor radius 11.3385 (-187.1104, -44.1624) -> (-175.7875, -54.9215) ccw
  circle A7 centre (5.5275, 51.8375) radius 1.2 construction
  circle A8 centre (-86.9725, 51.8375) radius 1.2 construction
  circle A9 centre (-179.5125, -51.1375) radius 1.2 construction
  circle A10 centre (-179.5125, 51.1375) radius 1.2 construction
  circle A11 centre (-120.5905, -51.9375) radius 1.2 construction
  circle A12 centre (-98.4725, -51.9375) radius 1.2 construction
  circle A13 centre (-23.2575, -51.9375) radius 1.2 construction
  circle A14 centre (8.8625, -51.8375) radius 1.2 construction
  circle A15 centre (13.6245, 51.8375) radius 1.2 construction
  circle A16 centre (179.6125, -51.8775) radius 1.2 construction
  circle A17 centre (94.2125, -51.7875) radius 1.2 construction
  circle A18 centre (180.1625, -0.1375) radius 1.2 construction
  circle A19 centre (96.7125, 51.6875) radius 1.2 construction
  circle A20 centre (179.5125, 52.1875) radius 1.2 construction
  line L10 (9.5245, 60.9965) -> (9.5245, 11.2835) construction
  arc A21 (7.5245, 9.2835) -> (9.5245, 11.2835) centre (7.5245, 11.2835) ccw construction
  line L11 (7.5245, 9.2835) -> (1.9995, 9.2835) construction
  arc A22 (1.9995, 9.2835) -> (-0.0005, 7.2835) centre (1.9995, 7.2835) ccw construction
  line L12 (-0.0005, 7.2835) -> (-0.0005, -7.7765) construction
  arc A23 (-2.0005, -9.7765) -> (-0.0005, -7.7765) centre (-2.0005, -7.7765) ccw construction
  line L13 (-2.0005, -9.7765) -> (-2.7625, -9.7765) construction
  arc A24 (-2.7625, -9.7765) -> (-4.7625, -11.7765) centre (-2.7625, -11.7765) ccw construction
  line L14 (-4.7625, -11.7765) -> (-4.7625, -26.8325) construction
  arc A25 (-4.7625, -26.8325) -> (-2.7625, -28.8325) centre (-2.7625, -26.8325) ccw construction
  line L15 (-2.7625, -28.8325) -> (2.7625, -28.8325) construction
  arc A26 (4.7625, -30.8325) -> (2.7625, -28.8325) centre (2.7625, -30.8325) ccw construction
  line L16 (4.7625, -30.8325) -> (4.7625, -54.9215) construction
  ellipse E2 centre (175.7875, -43.5674) end of major axis (175.7875, -54.9215) minor radius 11.3385 (175.7875, -54.9215) -> (187.1104, -44.1624) ccw
  line L17 (187.1104, -44.1624) -> (191.7393, 44.1624) construction
  ellipse E3 centre (175.7875, 45.0007) end of major axis (175.7875, 60.9965) minor radius 15.9738 (191.7393, 44.1624) -> (175.7875, 60.9965) ccw
  line L18 (175.7875, 60.9965) -> (9.5245, 60.9965) construction
  circle A27 centre (179.6125, -51.8775) radius 2.6
  circle A28 centre (94.2125, -51.7875) radius 2.6
  circle A29 centre (8.8625, -51.8375) radius 2.6
  circle A30 centre (0.7675, -51.9375) radius 2.6
  circle A31 centre (-23.2575, -51.9375) radius 2.6
  circle A32 centre (-98.4725, -51.9375) radius 2.6
  circle A33 centre (-120.5905, -51.9375) radius 2.6
  circle A34 centre (-179.5125, -51.1375) radius 2.6
  circle A35 centre (-179.5125, 51.1375) radius 2.6
  circle A36 centre (-86.9725, 51.8375) radius 2.6
  circle A37 centre (5.5275, 51.8375) radius 2.6
  circle A38 centre (13.6245, 51.8375) radius 2.6
  circle A39 centre (96.7125, 51.6875) radius 2.6
  circle A40 centre (179.5125, 52.1875) radius 2.6
  circle A41 centre (180.1625, -0.1375) radius 2.6
  line L19 (4.7625, -54.9215) -> (175.7875, -54.9215)
  dimension "d150" = 5.2
  constraint concentric A16 A27
  constraint concentric A17 A28
  constraint concentric A14 A29
  constraint concentric A0 A30
  constraint concentric A13 A31
  constraint concentric A12 A32
  constraint concentric A11 A33
  constraint concentric A9 A34
  constraint concentric A10 A35
  constraint concentric A8 A36
  constraint concentric A7 A37
  constraint concentric A15 A38
  constraint concentric A19 A39
  constraint concentric A20 A40
  constraint concentric A18 A41
  constraint equal A40 A41
  constraint equal A27 A40
  constraint equal A27 A28
  constraint equal A28 A39
  constraint equal A37 A39
  constraint equal A37 A38
  constraint equal A30 A38
  constraint equal A29 A30
  constraint equal A29 A31
  constraint equal A31 A32
  constraint equal A32 A33
  constraint equal A33 A34
  constraint equal A34 A35
  constraint equal A35 A36
  measures "d150" diameter of A35
ref_plane "WorkPlane8" through (184.2125, -8.4, -55.8375) normal (0, -1, 0) x (-1, 0, 0)
extrude "Extrude17" cut sketch "Sketch13" along normal blind 25 from surface at -11.6 bodies 3 8